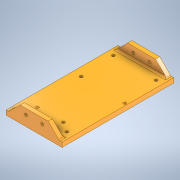
# Autodesk Inventor part: bottom_plate
Saved by Autodesk Inventor 2020 (Build 240168000, 168)
## iProperties
Created: 2021-04-04
Part Number: bottom_plate
Material: PET Plastic
Document SubType Name: Modeling
Designer: Devin
Density: 1.541 g/cm^3
Appearance: Smooth - Light Orange
Author: Devin
Autodesk Inventor part; units mm, degrees
ref_plane "YZ Plane" through (0, 0, 0) normal (1, 0, 0) x (0, 1, 0)
ref_plane "XZ Plane" through (0, 0, 0) normal (0, 1, 0) x (-1, 0, 0)
ref_plane "XY Plane" through (0, 0, 0) normal (0, 0, 1) x (1, 0, 0)
sketch "Sketch1" plane through (0, 0, 0) normal (0, 1, 0) x (-1, 0, 0)
  line L0 (0, 0) -> (60, 0)
  line L1 (60, 0) -> (60, -120)
  line L2 (60, -120) -> (0, -120)
  line L3 (0, -120) -> (0, 0)
  dimension "d0" = 60
  dimension "d1" = 120
  constraints: 8 end point, 2 parallel, 1 horizontal, 1 perpendicular
  measures "d0" distance of L0.start L0.end
  measures "d1" distance of L0.end L1.end
extrude "Extrusion1" add sketch "Sketch1" along normal blind 5
sketch "Sketch2" plane through (0, 5, 0) normal (0, 1, 0) x (1, 0, 0)
  line L0 (-30, 120) -> (-45, 120)
  line L1 (-30, 120) -> (-15, 120)
  line L2 (-45, 120) -> (-45, 115.5)
  line L3 (-45, 115.5) -> (-15, 115.5)
  line L4 (-15, 115.5) -> (-15, 120)
  line L5 (-15, 120) -> (-45, 120)
  line L6 (-60, 120) -> (-60, 0) projected
  line L7 (0, 0) -> (0, 120) projected
  line L8 (-30, 0) -> (-45, 0)
  line L9 (-30, 0) -> (-15, 0)
  line L10 (-45, 0) -> (-45, 4.5)
  line L11 (-45, 4.5) -> (-15, 4.5)
  line L12 (-15, 4.5) -> (-15, 0)
  line L13 (-45, 0) -> (-15, 0)
  line L14 (-60, 0) -> (0, 0) projected
  dimension "d9" = 15
  dimension "d10" = 15
  dimension "d12" = 4.5
  constraints: 24 end point, 2 parallel, 1 collinear, 1 perpendicular, 1 vertical
  measures "d9" distance of L0.start L0.end
  measures "d10" distance of L0.start L1.end
  measures "d12" distance of L0.end L2.end
extrude "Extrusion2" add sketch "Sketch2" along normal blind 12
chamfer "Chamfer1" distance 12 angle 45 4 edges at (-45, 5, -2.25) (-45, 5, -117.75) (-15, 5, -2.25) (-15, 5, -117.75)
fillet "Fillet1" radius 2 6 edges at (-30, 5, -115.5) (-56.9995, 5, -117.75) (-56.9995, 5, -2.25) (-30, 5, -4.5) (-3.0005, 5, -2.25) (-3.0005, 5, -117.75)
sketch "Sketch3" plane through (-60, 0, 0) normal (0, 0, 1) x (1, 0, 0)
  line L0 (0, 0) -> (60, 0) projected
  circle A0 centre (38.75, 11) radius 1.55
  circle A1 centre (21.25, 11) radius 1.55
  dimension "d22" = 3.1
  dimension "d23" = 3.1
  dimension "d25" = 17.5
  dimension "d26" = 11
  dimension "d27" = 11
  constraints: 2 centre point
  measures "d22" diameter of A0
  measures "d23" diameter of A1
  measures "d25" distance of A0.centre A1.centre
  measures "d26" distance from line of L0 A1.centre
  measures "d27" distance from line of L0 A0.centre
extrude "Extrusion3" cut sketch "Sketch3" against normal through all
sketch "Sketch4" plane through (0, 5, 0) normal (0, 1, 0) x (1, 0, 0)
  line L0 (0, 0) -> (0, 120) projected
  line L1 (0, 50.8517) -> (-60, 50.8517)
  line L2 (-60, 120) -> (-60, 0) projected
  line L3 (-26.65, 16.5517) -> (0, 16.5517)
  line L4 (0, 16.5517) -> (0, 85.1517)
  line L5 (0, 85.1517) -> (-53.3, 85.1517)
  line L6 (-53.3, 85.1517) -> (-53.3, 16.5517)
  line L7 (-53.3, 16.5517) -> (-26.65, 16.5517)
  line L8 (0, 85.1517) -> (0, 84.5517)
  line L9 (0, 85.1517) -> (0, 69.8517)
  circle A0 centre (-2.5, 69.8517) radius 1.55
  line L10 (-26.65, 85.1517) -> (-26.65, 16.5517)
  circle A1 centre (-50.7, 71.1517) radius 1.55
  circle A2 centre (-17.7, 19.0517) radius 1.55
  circle A3 centre (-45.6, 19.0517) radius 1.55
  line L11 (0, 85.1517) -> (-2, 85.1517)
  dimension "d34" = 53.3
  dimension "d35" = 68.6
  dimension "d39" = 3.1
  dimension "d43" = 3.1
  dimension "d44" = 3.1
  dimension "d55" = 14
  dimension "d56" = 1.3
  dimension "d57" = 50.8
  dimension "d58" = 15.2
  dimension "d59" = 27.9
  constraints: 20 end point, 4 centre point, 4 perpendicular, 3 point on line, 1 midpoint, 1 vertical
  measures "d34" distance of L4.end L5.end
  measures "d35" distance of L3.end L4.end
  measures "d39" diameter of A0
  measures "d43" diameter of A2
  measures "d44" diameter of A3
  measures "d55" distance from line of L5 A1.centre
  measures "d56" vertical distance of A0.centre A1.centre
  measures "d57" vertical distance of A2.centre A0.centre
  measures "d58" horizontal distance of A2.centre A0.centre
  measures "d59" distance of A3.centre A2.centre
extrude "Extrusion4" cut sketch "Sketch4" against normal blind 12 contours A0 | A1 | A2 | A3
sketch "Sketch5" plane through (0, 5, 0) normal (0, 1, 0) x (1, 0, 0)
  line L0 (0, 0) -> (0, 120) projected
  line L1 (0, 120) -> (0, 108)
  line L2 (0, 108) -> (-7, 108)
  line L3 (-60, 120) -> (-60, 0) projected
  circle A0 centre (-7, 108) radius 1.55
  line L4 (0, 120) -> (-60, 120) projected
  line L5 (-30, 120) -> (-30, 0)
  line L6 (-45, 0) -> (-15, 0) projected
  line L7 (0, 60) -> (-60, 60)
  circle A1 centre (-53, 108) radius 1.55
  circle A2 centre (-7, 12) radius 1.55
  circle A3 centre (-53, 12) radius 1.55
  dimension "d47" = 12
  dimension "d48" = 7
  dimension "d49" = 3.1
  constraints: 8 end point, 4 centre point, 4 midpoint, 3 symmetric about line, 1 coincident, 1 perpendicular, 1 point on line, 3 other
  measures "d47" distance of L0.end L1.end
  measures "d48" distance of L1.end L2.end
  measures "d49" diameter of A0
extrude "Extrusion5" cut sketch "Sketch5" against normal blind 10 contours A0 | A1 | A2 | A3
body "Solid1"
